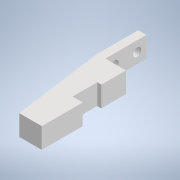
# Autodesk Inventor part: normal_finger
Saved by Autodesk Inventor 2021 (Build 250183000, 183)
## iProperties
Created: 2023-04-10
Part Number: normal_finger
Material: Generic
Document SubType Name: Modeling
Designer: mahmo
Density: 1 g/cm^3
Appearance: Default
Author: mahmo
Autodesk Inventor part; units mm, degrees
ref_plane "YZ Plane" through (0, 0, 0) normal (1, 0, 0) x (0, 1, 0)
ref_plane "XZ Plane" through (0, 0, 0) normal (0, 1, 0) x (-1, 0, 0)
ref_plane "XY Plane" through (0, 0, 0) normal (0, 0, 1) x (1, 0, 0)
sketch "Sketch1" plane through (0, 0, 0) normal (0, 1, 0) x (-1, 0, 0)
  line L0 (0, 0) -> (4, 0)
  line L1 (4, 0) -> (4, -20)
  line L2 (4, -20) -> (0, -20)
  line L3 (0, -20) -> (0, 0)
  line L4 (4, 0) -> (-10, 0)
  line L5 (-10, 0) -> (-10, 12)
  line L6 (-10, 12) -> (4, 12)
  line L7 (4, 12) -> (4, 0)
  line L8 (4, 12) -> (-8, 12)
  line L9 (-8, 12) -> (-8, 24)
  line L10 (-8, 24) -> (4, 24)
  line L11 (4, 24) -> (4, 12)
  line L12 (4, 24) -> (-6, 24)
  line L13 (-6, 24) -> (-6, 44)
  line L14 (-6, 44) -> (4, 44)
  line L15 (4, 44) -> (4, 24)
  line L16 (-2, 44) -> (4, 0)
  point P0 (-6, 24)
  dimension "d0" = 4
  dimension "d1" = 20
  dimension "d2" = 14
  dimension "d3" = 12
  dimension "d4" = 12
  dimension "d5" = 12
  dimension "d6" = 10
  dimension "d7" = 20
  constraints: 34 end point, 8 parallel, 4 horizontal, 4 perpendicular, 1 point on line
  measures "d0" distance of L1.end L2.end
  measures "d1" distance of L0.end L1.end
  measures "d2" distance of L5.end L6.end
  measures "d3" distance of L4.end L5.end
  measures "d4" distance of L9.end L10.end
  measures "d5" distance of L8.end L9.end
  measures "d6" distance of L13.end L14.end
  measures "d7" distance of L12.end L13.end
extrude "Extrusion1" add sketch "Sketch1" along normal blind 10 contours L4 L5 L6 L16 L0 | L0 L1 L2 L3 | L6 L9 L10 L16 | L10 L13 L14 L16
sketch "Sketch2" plane through (-4, 0, -20) normal (-1, 0, 0) x (0, 0, 1)
  circle A0 centre (15.5, 5) radius 2 projected
  circle A1 centre (4.5, 5) radius 2 projected
  point P0 (20, 0)
extrude "Extrusion2" cut sketch "Sketch2" against normal blind 10
move faces "Move1" translate (7, 0, 0) faces at (6, 6.6667, 37.3333)
move faces "Move2" translate (2, 0, 0) faces at (13, 6.6667, 37.3333)
move faces "Move3" translate (8, 0, 0) faces at (8, 6.6667, 20)
move faces "Move4" translate (7.75, 0, 0) faces at (10, 3.3333, 8)
sketch "Sketch3" plane through (0, 0, 0) normal (0, -1, 0) x (1, 0, 0)
  line L0 (12.2606, 4.3572) -> (4.6323, 4.3572)
  line L1 (4.6323, 4.3572) -> (4.6323, 40.636)
  line L2 (4.6323, 40.636) -> (12.2606, 40.636)
  line L3 (12.2606, 40.636) -> (12.2606, 4.3572)
  point P0 (0, 0)
  constraints: 8 end point, 2 parallel, 1 horizontal, 1 perpendicular
extrude "Extrusion3" cut sketch "Sketch3" against normal blind 10
move faces "Move5" translate (-0.5, 0, 0) faces at (12.2606, 3.3333, 16.4501)
fillet "Fillet1" radius 2 4 edges at (4.6323, 5, 4.3572) (4.6323, 5, 40.636) (11.7606, 5, 40.636) (11.7606, 5, 4.3572)
body "Solid1"
